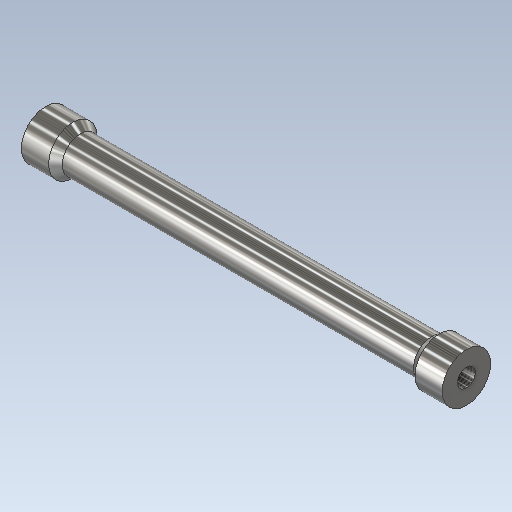
# Autodesk Inventor part: RCT-H010_Al_side_plate_post
Saved by Autodesk Inventor 2020 (Build 240168000, 168)
## iProperties
Created: 2019-09-18
Part Number: RCT-H010_Al_side_plate_post
Material: Generic
Document SubType Name: Modeling
Designer: maste
Density: 1 g/cm^3
Appearance: Default
Author: maste
Autodesk Inventor part; units mm, degrees
ref_plane "YZ Plane" through (0, 0, 0) normal (1, 0, 0) x (0, 1, 0)
ref_plane "XZ Plane" through (0, 0, 0) normal (0, 1, 0) x (-1, 0, 0)
ref_plane "XY Plane" through (0, 0, 0) normal (0, 0, 1) x (1, 0, 0)
sketch "Sketch1" plane through (0, 0, 0) normal (0, 0, 1) x (1, 0, 0)
  line L0 (-34.75, 0) -> (34.75, 0)
  line L1 (-34.75, 0) -> (-34.75, 4)
  line L2 (-34.75, 4) -> (-30.25, 4)
  line L3 (34.75, 0) -> (34.75, 4)
  line L4 (34.75, 4) -> (30.25, 4)
  line L5 (-29, 3) -> (29, 3)
  line L6 (-30.25, 4) -> (-29, 3)
  line L7 (30.25, 4) -> (29, 3)
  point P0 (0, 0)
  dimension "d0" = 69.5
  dimension "d1" = 0
  dimension "d2" = 34.75
  dimension "d3" = 4
  dimension "d4" = 4.5
  dimension "d5" = 4
  dimension "d6" = 4.5
  dimension "d7" = 58
  dimension "d8" = 3
  dimension "d9" = 29
  constraints: 16 end point, 2 horizontal, 2 perpendicular, 2 vertical
  measures "d0" distance of L0.start L0.end
  measures "d1" distance from line of point (0, 0) L0
  measures "d2" distance of point (0, 0) L0.start
  measures "d3" distance of L0.start L1.end
  measures "d4" distance of L1.end L2.end
  measures "d5" distance of L0.end L3.end
  measures "d6" distance of L3.end L4.end
  measures "d7" distance of L5.start L5.end
  measures "d8" distance between parallel lines of L0 L5
  measures "d9" horizontal distance of point (0, 0) L5.start
revolve "Revolution1" add sketch "Sketch1" angle 360 about axis through (-34.75, 0, 0) along (1, 0, 0)
sketch "Sketch2" plane through (34.75, 0, 0) normal (1, 0, 0) x (0, 0, -1)
  circle A0 centre (0, 0) radius 1.5
  dimension "d11" = 3
  constraints: 1 centre point, 1 coincident
  measures "d11" diameter of A0
extrude "Extrusion1" cut sketch "Sketch2" against normal blind 8
thread "Thread1" size "M3x0.5" class "6H" standard "ANSI Metric M Profile" full length
sketch "Sketch3" plane through (-34.75, 0, 0) normal (-1, 0, 0) x (0, 0, 1)
  circle A0 centre (0, 0) radius 1.5
  dimension "d16" = 3
  constraints: 1 centre point, 1 coincident
  measures "d16" diameter of A0
extrude "Extrusion2" cut sketch "Sketch3" against normal blind 8
thread "Thread2" size "M3x0.5" class "6H" standard "ANSI Metric M Profile" full length
body "Solid1"
